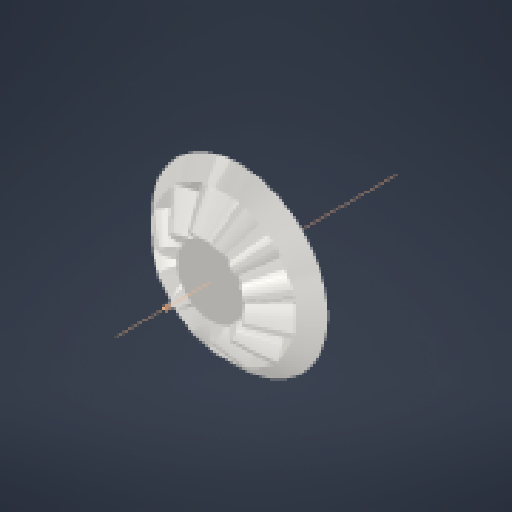
# Autodesk Inventor part: Engranaje biselado1
Saved by Autodesk Inventor 2026.2 (Build 302298010, 298A)
## iProperties
Created: 2026-04-17
Part Number: Engranaje biselado1
Material: Steel, Mild
Document SubType Name: Modeling
Designer: Jose Carlos
Categories: <?xml version="1.0" encoding="UTF-16"?> <MemberInstance><Categories><FamilyTemplate><FamilyTemplateParameter ValueType="xs:double" Id="1" ObjectReferenceKey="da_z" ObjectType="kUserParameterObject"/><FamilyTemplateParameter ValueType="xs:double" Id="2" ObjectReferenceKey="da_b" ObjectType="kUserParameterObject"/><FamilyTemplateParameter ValueType="xs:double" Id="3" ObjectReferenceKey="da_beta" ObjectType="kUserParameterObject"/><FamilyTemplateParameter ValueType="xs:double" Id="4" ObjectReferenceKey="da_dae" ObjectType="kUserParameterObject"/><FamilyTemplateParameter ValueType="xs:double" Id="5" ObjectReferenceKey="da_ve" ObjectType="kUserParameterObject"/><FamilyTemplateParameter ValueType="xs:double" Id="6" ObjectReferenceKey="da_omega" ObjectType="kUserParameterObject"/><FamilyTemplateParameter ValueType="xs:string" Id="7" ObjectReferenceKey="EAIAABAAAAAAHwAAAAAAAIAAAAAAAAAA" ObjectType="83914240" SubObjectId="SurfaceGeometry"/></FamilyTemplate><ParamToTemplateMap><ParamToTemplate CategoryParameter="//CategoryParameter[@InternalName='046C89C9-8512-4d59-83FE-43B91F4F132A']" TemplateParameter="1"/><ParamToTemplate CategoryParameter="//CategoryParameter[@InternalName='2552DF32-E462-4b46-AEBF-C6C7768E72AC']" TemplateParameter="2"/><ParamToTemplate CategoryParameter="//CategoryParameter[@InternalName='C9EE641D-15FC-4fae-A226-E94C4372FDD7']" TemplateParameter="3"/><ParamToTemplate><ParamToTemplate CategoryParameter="//CategoryParameter[@InternalName='00B6519A-459B-49c7-AD84-2E56D39A5744']" ConstantValue="0.000000"/></ParamToTemplate><ParamToTemplate><ParamToTemplate CategoryParameter="//CategoryParameter[@InternalName='04B31F0E-C7A6-4894-AA32-9629BEFACF47']" ConstantValue="1.000000"/></ParamToTemplate><ParamToTemplate><ParamToTemplate CategoryParameter="//CategoryParameter[@InternalName='43CBEC2E-7847-49e7-A936-2F7889FCB2D9']" ConstantValue="0.200000"/></ParamToTemplate><ParamToTemplate><ParamToTemplate CategoryParameter="//CategoryParameter[@InternalName='B1EFC894-105D-4ebd-86BF-FA20ED196853']" ConstantValue="0.300000"/></ParamToTemplate><ParamToTemplate><ParamToTemplate CategoryParameter="//CategoryParameter[@InternalName='51175063-3D10-4879-93E8-6246FE8B403D']" ConstantValue="2060000000.000000"/></ParamToTemplate><ParamToTemplate><ParamToTemplate CategoryParameter="//CategoryParameter[@InternalName='A3A52E27-4454-46a9-B0BD-C932399B70AF']" ConstantValue="0.300000"/></ParamToTemplate><ParamToTemplate CategoryParameter="//CategoryParameter[@InternalName='2A200944-5A8C-41ca-B96E-8520D2E510F1']" TemplateParameter="4"/><ParamToTemplate><ParamToTemplate CategoryParameter="//CategoryParameter[@InternalName='1A637F62-92C8-44bc-B81F-10802510B579']" ConstantValue="1.221616"/></ParamToTemplate><ParamToTemplate CategoryParameter="//CategoryParameter[@InternalName='B52DD4BE-6863-48fb-BF58-89EF6F9EC65C']" TemplateParameter="5"/><ParamToTemplate><ParamToTemplate CategoryParameter="//CategoryParameter[@InternalName='3956BFF2-84D2-457d-93C2-9B0613DEBA67']" ConstantValue="0.482085"/></ParamToTemplate><ParamToTemplate CategoryParameter="//CategoryParameter[@InternalName='739CFA02-461B-4bf8-8049-181FCAD8B28F']" TemplateParameter="6"/><ParamToTemplate><ParamToTemplate CategoryParameter="//CategoryParameter[@InternalName='A27E999F-E2CE-4481-8A2A-EBF499C4C3C5']" ConstantValue="0.000000"/></ParamToTemplate><ParamToTemplate><ParamToTemplate CategoryParameter="//CategoryParameter[@InternalName='9E1B4470-B2D3-4ff1-B813-535BB4CDF51A']" ConstantValue="3520000.000000"/></ParamToTemplate><ParamToTemplate><ParamToTemplate CategoryParameter="//CategoryParameter[@InternalName='F8452263-BFF6-458c-9FB1-07C4B99E95CD']" ConstantValue="11400000.000000"/></ParamToTemplate><ParamToTemplate><ParamToTemplate CategoryParameter="//CategoryParameter[@InternalName='3E3BB259-FD49-497f-8171-6EBC954A3479']" ConstantValue="2.000000"/></ParamToTemplate><ParamToTemplate CategoryParameter="//CategoryParameter[@InternalName='27C3BAF2-7550-4e4b-AE2C-0DB134B7D9B7']" TemplateParameter="7"/></ParamToTemplateMap><Category DisplayName="Gear" InternalName="DC85795E-93AB-48d5-8EEE-5A27447B64BD" Mnemonic="Gear"><CategoryParameter DisplayName="z" InternalName="046C89C9-8512-4d59-83FE-43B91F4F132A" Mnemonic="z"/><CategoryParameter DisplayName="b" InternalName="2552DF32-E462-4b46-AEBF-C6C7768E72AC" Mnemonic="b"/><CategoryParameter DisplayName="||b|" InternalName="C9EE641D-15FC-4fae-A226-E94C4372FDD7" Mnemonic="beta"/><CategoryParameter DisplayName="x" InternalName="00B6519A-459B-49c7-AD84-2E56D39A5744" Mnemonic="x"/><CategoryParameter DisplayName="a*" InternalName="04B31F0E-C7A6-4894-AA32-9629BEFACF47" Mnemonic="a"/><CategoryParameter DisplayName="c*" InternalName="43CBEC2E-7847-49e7-A936-2F7889FCB2D9" Mnemonic="c"/><CategoryParameter DisplayName="r|.f|*" InternalName="B1EFC894-105D-4ebd-86BF-FA20ED196853" Mnemonic="rf"/><CategoryParameter DisplayName="E" InternalName="51175063-3D10-4879-93E8-6246FE8B403D" Mnemonic="E"/><CategoryParameter DisplayName="||m|" InternalName="A3A52E27-4454-46a9-B0BD-C932399B70AF" Mnemonic="mi"/><Category DisplayName="BevelGear" InternalName="0C98F69A-0C2B-4791-B2FE-7691BB227E77" Mnemonic="BevelGear"><CategoryParameter DisplayName="d|.ae|" InternalName="2A200944-5A8C-41ca-B96E-8520D2E510F1" Mnemonic="dae"/><CategoryParameter DisplayName="d|.ai|" InternalName="1A637F62-92C8-44bc-B81F-10802510B579" Mnemonic="dai"/><CategoryParameter DisplayName="A|.e|" InternalName="B52DD4BE-6863-48fb-BF58-89EF6F9EC65C" Mnemonic="ve"/><CategoryParameter DisplayName="A|.i|" InternalName="3956BFF2-84D2-457d-93C2-9B0613DEBA67" Mnemonic="vi"/><CategoryParameter DisplayName="||S|" InternalName="739CFA02-461B-4bf8-8049-181FCAD8B28F" Mnemonic="omega"/><CategoryParameter DisplayName="x|.t|" InternalName="A27E999F-E2CE-4481-8A2A-EBF499C4C3C5" Mnemonic="xt"/><CategoryParameter DisplayName="||s||.Flim|" InternalName="9E1B4470-B2D3-4ff1-B813-535BB4CDF51A" Mnemonic="sFlim"/><CategoryParameter DisplayName="||s||.Hlim|" InternalName="F8452263-BFF6-458c-9FB1-07C4B99E95CD" Mnemonic="sHlim"/><CategoryParameter DisplayName="tipo" InternalName="3E3BB259-FD49-497f-8171-6EBC954A3479" Mnemonic="type"/><CategoryParameter DisplayName="PitchDiameter" InternalName="27C3BAF2-7550-4e4b-AE2C-0DB134B7D9B7" Mnemonic="IDS_PITCHDIAM"/></Category></Category></Categories></MemberInstance>
Mass: 60.9118 g
Surface Area: 34.3074 cm^2
Volume: 7.7496 cm^3
Density: 7.86 g/cm^3
Appearance: Steel
CustomPartVersion: 1
Author: Jose Carlos
Autodesk Inventor part; units mm, degrees
ref_plane "Plano de malla 2" through (0, 0, 0) normal (0.9659258, 0.258819, 0) x (0, 0, 1)
sketch "Boceto de cuerpo dentado" plane through (0, 0, 0) normal (1, 0, 0) x (0, 1, 0)
  line L0 (0, 0) -> (7.7272, -10.2728) construction
  line L1 (7.7272, -10.2728) -> (10.06, -7.94)
  line L2 (10.06, -7.94) -> (0, 0) construction
  line L3 (9, -9) -> (0, 0) construction
  line L4 (4.6917, -6.2373) -> (6.1081, -4.8209)
  line L5 (7.7272, -10.2728) -> (4.6917, -6.2373)
  line L6 (10.06, -7.94) -> (6.1081, -4.8209)
  line L7 (0, -12.3274) -> (0, 2.0546) projected
  line L8 (0, -9) -> (10.06, -9) construction
  line L9 (7.7272, -10.2728) -> (12.3929, -10.2728)
  line L10 (12.3929, -10.2728) -> (10.06, -7.94)
  dimension "d0" = 18
  dimension "d1" = 15.4544
  dimension "d2" = 20.1201
  dimension "d3" = 5
  dimension "d4" = 7.94
  constraints: 20 end point, 4 perpendicular, 4 point on line, 2 collinear, 1 horizontal, 1 horizontal alignment, 1 vertical alignment
  measures "d0" diameter of L3.start L7
  measures "d1" diameter of L0.end L7
  measures "d2" diameter of L1.end L7
  measures "d3" distance between parallel lines of L1 L4
  measures "d4" vertical distance of L1.end L0.start
revolve "Cuerpo dentado" add sketch "Boceto de cuerpo dentado" angle 360 about axis through (0, 0, 0) along (0, 0, 1)
ref_plane "Plano de diente" through (0, 9, -9) normal (0, -0.7071068, 0.7071068) x (1, 0, 0)
sketch "Boceto inicial" plane through (0, 9, -9) normal (0, -0.7071068, 0.7071068) x (1, 0, 0)
  line L0 (0, -15.7719) -> (0, 5.5357) projected
  arc A0 (-0.6816, -2.1959) -> (-3.3488, 2.1158) centre (-5.5345, -2.2171) ccw
  arc A1 (3.3488, 2.1158) -> (0.6816, -2.1959) centre (5.5345, -2.2171) ccw
  line L1 (-0.6816, -2.1959) -> (0.6816, -2.1959)
  arc A2 (3.3488, 2.1158) -> (-3.3488, 2.1158) centre (0, -12.7279) ccw
  dimension "d7" = 4.853
  dimension "d8" = 5.5345
  dimension "d9" = 10.5108
  dimension "d57" = 15.2168
  dimension "d58" = 10.532
  constraints: 6 point on circle, 3 centre point, 3 symmetric about line, 2 end point, 1 coincident, 1 perpendicular, 1 other
  measures "d7" radius of A0
  measures "d8" horizontal distance of point (0, -12.728) A0.centre
  measures "d9" vertical distance of point (0, -12.728) A0.centre
  measures "d57" radius of A2
  measures "d58" distance from line of A2.centre L1
ref_plane "Plano final" through (0, 5.3478, -5.3478) normal (0, -0.7071068, 0.7071068) x (1, 0, 0)
sketch "Boceto final" plane through (0, 5.3478, -5.3478) normal (0, -0.7071068, 0.7071068) x (1, 0, 0)
  line L0 (0, -9.3717) -> (0, 3.2893) projected
  arc A0 (-0.405, -1.3048) -> (-1.9899, 1.2572) centre (-3.2886, -1.3174) ccw
  arc A1 (1.9899, 1.2572) -> (0.405, -1.3048) centre (3.2886, -1.3174) ccw
  line L1 (-0.405, -1.3048) -> (0.405, -1.3048)
  arc A2 (1.9899, 1.2572) -> (-1.9899, 1.2572) centre (0, -7.563) ccw
  dimension "d12" = 2.8836
  dimension "d15" = 3.2886
  dimension "d16" = 6.2456
  dimension "d59" = 9.0419
  dimension "d60" = 6.2582
  constraints: 6 point on circle, 3 centre point, 3 symmetric about line, 2 end point, 1 coincident, 1 other
  measures "d12" radius of A0
  measures "d15" horizontal distance of A0.centre point (0, -7.563)
  measures "d16" vertical distance of A0.centre point (0, -7.563)
  measures "d59" radius of A2
  measures "d60" distance from line of A2.centre L1
loft "Loft" cut profiles "Boceto inicial", "Boceto final"
pattern_circular "Circular Pattern" count 12 over 360 about axis through (0, 0, 0) along (0, 0, 1) of "Loft"
sketch3d "Boceto 3D derecho"
ref_plane "Plano final derecho" through (-1.3745, 5.1682, -5.3478) normal (0.1817371, -0.6833532, 0.7071068) x (0.9664074, 0.257015, 0)
sketch "Boceto final derecho" plane through (-1.3745, 5.1682, -5.3478) normal (0.1817371, -0.6833532, 0.7071068) x (0.9664074, 0.257015, 0)
  arc A0 (-0.405, -1.3048) -> (-1.9899, 1.2572) centre (-3.2886, -1.3174) ccw
  line L0 (0, -10.9889) -> (0, 4.9066) projected
  arc A1 (1.9899, 1.2572) -> (0.405, -1.3048) centre (3.2886, -1.3174) ccw
  line L1 (-0.405, -1.3048) -> (0.405, -1.3048)
  arc A2 (1.9899, 1.2572) -> (-1.9899, 1.2572) centre (0, -7.563) ccw
  dimension "d70" = 3.2886
  dimension "d71" = 6.2456
  dimension "d72" = 2.8836
  dimension "d73" = 6.2582
  dimension "d74" = 9.0419
  constraints: 6 point on circle, 3 centre point, 3 symmetric about line, 2 end point, 1 coincident, 1 perpendicular, 1 other
  measures "d70" horizontal distance of A2.centre A0.centre
  measures "d71" vertical distance of point (0, -7.563) A0.centre
  measures "d72" radius of A0
  measures "d73" distance from line of point (0, -7.563) L1
  measures "d74" radius of A2
feature "Solevación derecha" [suppressed]
pattern_circular "Patrón circular derecho" [suppressed]
sketch3d "Boceto 3D izquierdo"
ref_plane "Plano final izquierdo" through (1.378, 5.1682, -5.3492) normal (-0.1821641, -0.6832108, 0.7071346) x (0.9662439, -0.257629, 0)
sketch "Boceto final izquierdo" plane through (1.378, 5.1682, -5.3492) normal (-0.1821641, -0.6832108, 0.7071346) x (0.9662439, -0.257629, 0)
  line L0 (0, -12.5803) -> (0, 6.3333) projected
  arc A0 (-0.405, -1.3045) -> (-1.9899, 1.2575) centre (-3.2886, -1.3171) ccw
  arc A1 (1.9899, 1.2575) -> (0.405, -1.3045) centre (3.2886, -1.3171) ccw
  line L1 (-0.405, -1.3045) -> (0.405, -1.3045)
  ellipse E0 centre (0, -3.4087) end of major axis (6.1081, -3.4087) minor radius 4.3192 projected
  arc A2 (1.9899, 1.2575) -> (-1.9899, 1.2575) centre (0, -7.5627) ccw
  point P0 (0, -7.5627)
  dimension "d56" = 4.3192
  dimension "d30" = 2.8836
  dimension "d31" = 3.2886
  dimension "d32" = 6.2456
  dimension "d61" = 9.0419
  dimension "d62" = 6.2582
  constraints: 6 point on circle, 3 centre point, 3 symmetric about line, 2 end point, 1 coincident, 2 other
  measures "d30" radius of A0
  measures "d31" horizontal distance of point (0, -7.563) A0.centre
  measures "d32" vertical distance of A0.centre point (0, -7.563)
  measures "d61" radius of A2
  measures "d62" distance from line of point (0, -7.563) L1
feature "Solevación izquierda" [suppressed]
pattern_circular "Patrón circular izquierdo" [suppressed]
sketch "Boceto de cuerpo" plane through (0, 0, 0) normal (1, 0, 0) x (0, 1, 0)
  line L0 (0, -11.0799) -> (0, -5.4302) projected
  line L1 (7.7272, -10.2728) -> (4.6917, -6.2373) projected
  line L2 (4.6917, -6.2373) -> (0, -6.2373)
  line L3 (7.7272, -10.2728) -> (0, -10.2728)
  constraints: 4 end point, 2 perpendicular, 2 point on line
revolve "Fijar cuerpo" add sketch "Boceto de cuerpo" angle 360 about axis through (0, 0, 0) along (0, 0, 1)
sketch "Sketch6" plane through (0, 0, 0) normal (1, 0, 0) x (0, 1, 0)
  line L0 (9, -9) -> (0, 0) projected
  line L1 (0, -10.8) -> (0, 1.8) projected
surface revolve "Diámetro de separación" sketch "Sketch6" angle 360 about axis through (0, 0, 0) along (0, 0, 1) shown no curves L0
equation "\"d0\" = da_de"
equation "\"d1\" = da_dfe"
equation "\"d2\" = da_dae"
equation "\"d3\" = da_b"
equation "\"d4\" = da_ve"
equation "\"d7\" = fd_rr"
equation "\"d8\" = fd_x"
equation "\"d9\" = fd_y"
equation "\"d57\" = 0.5 * fd_dva + 0.3 * da_he"
equation "\"d58\" = 0.5 * fd_dva - 1.12 * da_he"
equation "\"da_teethtype\" = 0"
equation "\"da_b\" = 5"
equation "\"da_de\" = 18"
equation "\"da_dae\" = 20.12007"
equation "\"da_dfe\" = 15.45442"
equation "\"da_le\" = 12.72792"
equation "\"da_omega\" = 90deg"
equation "\"da_beta\" = 0"
equation "\"da_delta\" = 45deg"
equation "\"da_alpha\" = 20deg"
equation "\"da_he\" = 3.29912"
equation "\"da_ve\" = 7.93996"
equation "\"da_zv\" = 16.970563"
equation "\"fd_loft\" = da_b + 0.05 * da_he"
equation "\"fd_x\" = fd_x1 + fd_x2"
equation "\"fd_y\" = fd_y1 - fd_y2"
equation "\"fd_dd\" = fd_dva - 0.8 * da_he"
equation "\"da_dvw\" = 25.45584"
equation "\"d11\" = fd_loft"
equation "\"da_dm\" = 14.46447"
equation "\"da_x\" = 0"
equation "\"da_m\" = 1.5"
equation "\"d50\" = da_omega"
equation "\"fd_rr\" = 4.852955"
equation "\"fd_dva\" = 28.454078"
equation "\"fd_x1\" = 1.189449"
equation "\"fd_x2\" = 4.345067"
equation "\"fd_y1\" = 12.672222"
equation "\"fd_y2\" = 2.161381"
body "Solid1"
body "Srf1"
